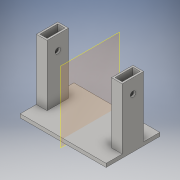
# Autodesk Inventor part: MiddlePostsForTwoSprockets
Saved by Autodesk Inventor 2016 SP1 (Build 200210100, 210)
## iProperties
Created: 2016-02-12
Part Number: MiddlePostsForTwoSprockets
Material: Generic
Document SubType Name: Modeling
Designer: steele
Density: 1 g/cm^3
Appearance: Default
Author: steele
Autodesk Inventor part; units mm, degrees
ref_plane "XZ Plane" through (0, 0, 0) normal (0, 1, 0) x (-1, 0, 0)
ref_plane "XY Plane" through (0, 0, 0) normal (0, 0, 1) x (1, 0, 0)
sketch "Sketch1" plane through (0, 0, 0) normal (0, 1, 0) x (-1, 0, 0)
  line L0 (76.2, 47.625) -> (-76.2, 47.625)
  line L1 (-76.2, 47.625) -> (-76.2, -47.625)
  line L2 (-76.2, -47.625) -> (76.2, -47.625)
  line L3 (76.2, -47.625) -> (76.2, 47.625)
  line L4 (76.2, 47.625) -> (-76.2, -47.625) construction
  line L5 (-76.2, 47.625) -> (76.2, -47.625) construction
  point P0 (0, 0)
  dimension "d0" = 152.4
  dimension "d1" = 95.25
  constraints: 12 end point, 2 midpoint, 2 parallel, 1 horizontal, 1 perpendicular
  measures "d0" distance of L0.start L0.end
  measures "d1" distance of L2.end L0.start
extrude "Extrusion1" add sketch "Sketch1" against normal blind 6.35
sketch "Sketch4" plane through (0, 0, 0) normal (0, 1, 0) x (1, 0, 0)
  line L0 (-76.2, -19.05) -> (-57.15, -19.05)
  line L1 (-57.15, -19.05) -> (-57.15, 19.05)
  line L2 (-57.15, 19.05) -> (-76.2, 19.05)
  line L3 (-76.2, 19.05) -> (-76.2, -19.05)
  line L4 (-76.2, -19.05) -> (-57.15, 19.05) construction
  line L5 (-57.15, -19.05) -> (-76.2, 19.05) construction
  line L6 (-76.2, 47.625) -> (-76.2, -47.625) projected
  line L7 (-73.025, -15.875) -> (-60.325, -15.875)
  line L8 (-60.325, -15.875) -> (-60.325, 15.875)
  line L9 (-60.325, 15.875) -> (-73.025, 15.875)
  line L10 (-73.025, 15.875) -> (-73.025, -15.875)
  line L11 (-73.025, -15.875) -> (-60.325, 15.875) construction
  line L12 (-60.325, -15.875) -> (-73.025, 15.875) construction
  point P0 (0, 0)
  point P1 (-66.675, 0)
  dimension "d8" = 0
  dimension "d9" = 38.1
  dimension "d10" = 19.05
  dimension "d11" = 3.175
  dimension "d12" = 3.175
  constraints: 24 end point, 4 midpoint, 4 parallel, 2 horizontal, 2 perpendicular, 1 collinear
  measures "d8" vertical distance of point (0, 0) point (-66.675, 0)
  measures "d9" distance of L0.end L1.end
  measures "d10" distance of L0.start L0.end
  measures "d11" distance between parallel lines of L3 L10
  measures "d12" distance between parallel lines of L0 L7
extrude "Extrusion2" add sketch "Sketch4" along normal blind 107.95
sketch "Sketch5" plane through (-76.2, -6.35, -47.625) normal (-1, 0, 0) x (0, 0, 1)
  circle A0 centre (47.625, 88.9) radius 4.7625
  line L0 (28.575, 114.3) -> (66.675, 114.3) projected
  line L1 (47.625, 6.35) -> (47.625, 114.3) construction
  dimension "d15" = 9.525
  dimension "d16" = 25.4
  dimension "d19" = 0
  constraints: 2 end point, 1 centre point, 1 midpoint
  measures "d15" diameter of A0
  measures "d16" distance from line of A0.centre L0
  measures "d19" distance from line of A0.centre L1
extrude "Extrusion3" cut sketch "Sketch5" against normal through all
mirror "Mirror1" about plane through (0, 0, 0) normal (1, 0, 0) of "Extrusion2", "Extrusion3"
equation "\"d0\" = baseWidth"
equation "\"d1\" = baseLength"
equation "\"d2\" = baseThickness"
equation "\"d9\" = postLength"
equation "\"d10\" = postWidth"
equation "\"d11\" = postWallThickness"
equation "\"d12\" = postWallThickness"
equation "\"d13\" = postHeight"
equation "\"d15\" = postAxelDiam"
equation "\"d16\" = heightFromTopToAxelCenter"
equation "\"d17\" = postHeight"
equation "\"baseWidth\" = 152.4"
equation "\"baseLength\" = 95.25"
equation "\"baseThickness\" = 6.35"
equation "\"postWidth\" = 19.05"
equation "\"postLength\" = 38.1"
equation "\"postWallThickness\" = 3.175"
equation "\"postAxelDiam\" = 9.525"
equation "\"heightFromTopToAxelCenter\" = 25.4"
equation "\"diamOfSproketPlusChain\" = 152.4"
equation "\"radiusOfSprocket\" = 0.5 * diamOfSproketPlusChain"
equation "\"heightOfAxelAboveBasePlate\" = radiusOfSprocket + gapBetweenChainAndBasePlate"
equation "\"gapBetweenChainAndBasePlate\" = 6.35"
equation "\"heightAboveRobotPlate\" = 50.8"
equation "\"postHeight\" = 107.95"
body "Solid1"
